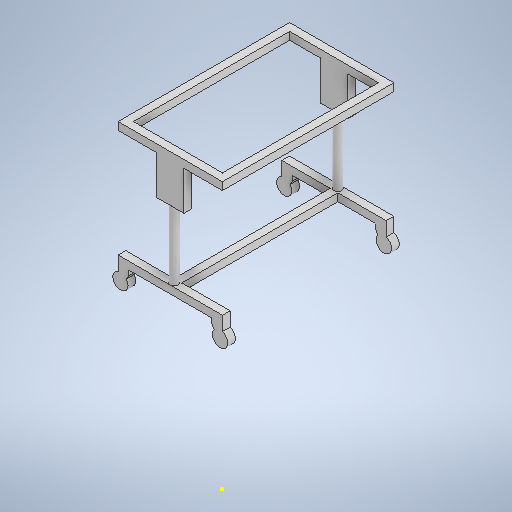
# Autodesk Inventor part: Human-Subject-Cart
Saved by Autodesk Inventor 2025.1 (Build 291241000, 241)
## iProperties
Created: 2025-01-22
Part Number: Human-Subject-Cart
Material: Generic
Document SubType Name: Modeling
Designer: jmarvel
Density: 1 g/cm^3
Appearance: Default
Author: jmarvel
Autodesk Inventor part; units mm, degrees
ref_plane "YZ Plane" through (0, 0, 0) normal (1, 0, 0) x (0, 1, 0)
ref_plane "XZ Plane" through (0, 0, 0) normal (0, 1, 0) x (-1, 0, 0)
ref_plane "XY Plane" through (0, 0, 0) normal (0, 0, 1) x (1, 0, 0)
sketch "Sketch1" plane through (0, 0, 0) normal (0, 1, 0) x (-1, 0, 0)
  line L0 (0, 0) -> (680, 0)
  line L1 (680, 0) -> (680, -1118)
  line L2 (680, -1118) -> (0, -1118)
  line L3 (0, -1118) -> (0, 0)
  dimension "d0" = 680
  dimension "d1" = 1118
  constraints: 8 end point, 2 parallel, 1 horizontal, 1 perpendicular
  measures "d0" distance of L1.end L2.end
  measures "d1" distance of L0.end L1.end
extrude "Extrusion1" add sketch "Sketch1" along normal blind 50
sketch "Sketch2" plane through (0, 50, 0) normal (0, 1, 0) x (1, 0, 0)
  line L0 (-50, 50) -> (-630, 50)
  line L1 (-630, 50) -> (-630, 1068)
  line L2 (-630, 1068) -> (-50, 1068)
  line L3 (-50, 1068) -> (-50, 50)
  point P0 (0, 0)
  dimension "d4" = 580
  dimension "d5" = 1018
  constraints: 8 end point, 2 parallel, 1 horizontal, 1 perpendicular
  measures "d4" distance of L1.end L2.end
  measures "d5" distance of L0.end L1.end
extrude "Extrusion2" cut sketch "Sketch2" against normal blind 50
sketch "Sketch3" plane through (0, 50, 0) normal (0, 1, 0) x (1, 0, 0)
  point P0 (0, 0)
sketch "Sketch4" plane through (0, 50, 0) normal (0, 1, 0) x (1, 0, 0)
  line L0 (-680, 0) -> (0, 0) projected
  line L1 (-251, 0) -> (-429, 0)
  line L2 (-429, 0) -> (-429, 50)
  line L3 (-429, 50) -> (-251, 50)
  line L4 (-251, 50) -> (-251, 0)
  dimension "d8" = 178
  dimension "d9" = 50
  constraints: 8 end point, 2 parallel, 1 horizontal, 1 perpendicular, 1 point on line
  measures "d8" distance of L2.end L3.end
  measures "d9" distance of L1.end L2.end
extrude "Extrusion3" add sketch "Sketch4" along normal blind 254
sketch "Sketch5" plane through (0, 50, 0) normal (0, 1, 0) x (1, 0, 0)
  line L0 (0, 1118) -> (-680, 1118) projected
  line L1 (-630, 1068) -> (-50, 1068) projected
  line L2 (-251, 1118) -> (-429, 1118)
  line L3 (-429, 1118) -> (-429, 1068)
  line L4 (-429, 1068) -> (-251, 1068)
  line L5 (-251, 1068) -> (-251, 1118)
  point P0 (0, 0)
  dimension "d12" = 178
  constraints: 8 end point, 2 parallel, 2 point on line, 1 horizontal, 1 perpendicular
  measures "d12" distance of L4.end L3.end
extrude "Extrusion4" add sketch "Sketch5" along normal blind 254
sketch "Sketch6" plane through (0, 304, 0) normal (0, 1, 0) x (1, 0, 0)
  circle A0 centre (-340, 25) radius 25
  point P0 (0, 0)
  dimension "d15" = 50
  constraints: 1 centre point
  measures "d15" diameter of A0
extrude "Extrusion5" add sketch "Sketch6" along normal blind 450
sketch "Sketch7" plane through (0, 304, 0) normal (0, 1, 0) x (1, 0, 0)
  circle A0 centre (-340, 1093) radius 25
  point P0 (0, 0)
  dimension "d18" = 50
  constraints: 1 centre point
  measures "d18" diameter of A0
extrude "Extrusion6" add sketch "Sketch7" along normal blind 450
sketch "Sketch8" plane through (-340, 754, -25) normal (0, 1, 0) x (1, 0, 0)
  line L0 (-340, -25) -> (340, -25) projected
  line L1 (25, -25) -> (-25, -25)
  line L2 (-25, -25) -> (-25, 1093)
  line L3 (-25, 1093) -> (25, 1093)
  line L4 (25, 1093) -> (25, -25)
  dimension "d21" = 50
  dimension "d22" = 1118
  constraints: 8 end point, 2 parallel, 1 horizontal, 1 perpendicular, 1 point on line
  measures "d21" distance of L2.end L3.end
  measures "d22" distance of L1.end L2.end
extrude "Extrusion7" add sketch "Sketch8" along normal blind 50
sketch "Sketch9" plane through (-315, 754, -25) normal (1, 0, 0) x (0, 0, -1)
  line L0 (0, 0) -> (-25, 0) projected
  line L1 (-25, 0) -> (25, 0)
  line L2 (25, 0) -> (25, 50)
  line L3 (25, 50) -> (-25, 50)
  line L4 (-25, 50) -> (-25, 0)
  point P0 (-25, -754)
  dimension "d25" = 50
  dimension "d26" = 50
  constraints: 8 end point, 2 parallel, 1 horizontal, 1 perpendicular
  measures "d25" distance of L3.end L2.end
  measures "d26" distance of L2.end L1.end
extrude "Extrusion8" add sketch "Sketch9" along normal blind 315
sketch "Sketch10" plane through (-315, 754, -1093) normal (1, 0, 0) x (0, 0, -1)
  line L0 (25, 0) -> (25, 50) projected
  line L1 (25, 0) -> (-25, 0)
  line L2 (-25, 0) -> (-25, 50)
  line L3 (-25, 50) -> (25, 50)
  line L4 (25, 50) -> (25, 0)
  point P0 (-1093, -754)
  dimension "d29" = 50
  dimension "d30" = 50
  constraints: 8 end point, 2 parallel, 1 horizontal, 1 perpendicular
  measures "d29" distance of L2.end L3.end
  measures "d30" distance of L1.end L2.end
extrude "Extrusion9" add sketch "Sketch10" along normal blind 315
sketch "Sketch11" plane through (-365, 754, -1093) normal (-1, 0, 0) x (0, 0, 1)
  line L0 (-25, 50) -> (1093, 50) projected
  line L1 (-25, 50) -> (25, 50)
  line L2 (25, 50) -> (25, 0)
  line L3 (25, 0) -> (-25, 0)
  line L4 (-25, 0) -> (-25, 50)
  point P0 (1093, -754)
  dimension "d33" = 50
  dimension "d34" = 50
  constraints: 8 end point, 2 parallel, 1 horizontal, 1 perpendicular
  measures "d33" distance of L2.end L3.end
  measures "d34" distance of L1.end L2.end
extrude "Extrusion10" add sketch "Sketch11" along normal blind 315
sketch "Sketch12" plane through (-365, 754, -25) normal (-1, 0, 0) x (0, 0, 1)
  line L0 (-1043, 50) -> (25, 50) projected
  line L1 (25, 50) -> (-25, 50)
  line L2 (-25, 50) -> (-25, 0)
  line L3 (-25, 0) -> (25, 0)
  line L4 (25, 0) -> (25, 50)
  point P0 (25, -754)
  dimension "d37" = 50
  dimension "d38" = 50
  constraints: 8 end point, 2 parallel, 1 horizontal, 1 perpendicular
  measures "d37" distance of L3.end L2.end
  measures "d38" distance of L2.end L1.end
extrude "Extrusion11" add sketch "Sketch12" along normal blind 315
sketch "Sketch13" plane through (0, 754, -1118) normal (0, 0, -1) x (-1, 0, 0)
  line L0 (680, 0) -> (680, 50) projected
  line L1 (680, 50) -> (610, 50)
  line L2 (610, 50) -> (610, 80.718)
  line L3 (650, 150) -> (680, 150)
  line L4 (680, 150) -> (680, 50)
  line L5 (0, 50) -> (70, 50)
  line L6 (70, 50) -> (70, 80.718)
  line L7 (30, 150) -> (0, 150)
  line L8 (0, 150) -> (0, 50)
  line L9 (650, 150) -> (610, 80.718)
  line L10 (650, 150) -> (680, 150) construction
  line L11 (30, 150) -> (70, 80.718)
  point P0 (0, -754)
  constraints: 22 end point, 4 parallel, 3 horizontal, 2 perpendicular, 1 point on line
extrude "Extrusion12" add sketch "Sketch13" against normal blind 1118
sketch "Sketch14" plane through (0, 754, -25) normal (1, 0, 0) x (0, 0, -1)
  line L0 (25, 50) -> (1043, 50) projected
  line L1 (1043, 50) -> (25, 50)
  line L2 (25, 50) -> (25, 150)
  line L3 (25, 150) -> (1043, 150)
  line L4 (1043, 150) -> (1043, 50)
  point P0 (-25, -754)
  constraints: 8 end point, 2 parallel, 1 horizontal, 1 perpendicular
extrude "Extrusion13" cut sketch "Sketch14" against normal blind 1118
sketch "Sketch15" plane through (-340, 754, 0) normal (0, 0, 1) x (1, 0, 0)
  circle A0 centre (325, 140) radius 50
  circle A1 centre (-325, 140) radius 50
  line L0 (340, 0) -> (340, 150) projected
  line L1 (340, 0) -> (340, 150) projected
  line L2 (0, 0) -> (-340, 0) projected
  line L3 (0, 0) -> (340, 0) projected
  line L4 (340, 0) -> (340, 150) projected
  line L5 (340, 150) -> (310, 150) projected
  line L6 (310, 150) -> (270, 80.718) projected
  line L7 (270, 80.718) -> (270, 50) projected
  line L8 (270, 50) -> (-270, 50) projected
  line L9 (-270, 50) -> (-270, 80.718) projected
  line L10 (-270, 80.718) -> (-310, 150) projected
  line L11 (-310, 150) -> (-340, 150) projected
  line L12 (-340, 0) -> (-340, 150) projected
  point P0 (340, -754)
  point P1 (340, 92.303)
  point P2 (286.0942, 108.594)
  constraints: 2 centre point
extrude "Extrusion14" add sketch "Sketch15" against normal blind 1118 contours A0 L0 L5 L6 | L12 L11 L10 A1 | A1 L10 L11 L12 picked at (325.7082, 163.3183)
move or copy body "Rotate1" bodies to move or copy 1 copy no rotation origin (0, 0, 0) rotation axis (1, 0, 0) rotation angle 180 translate (0, 1788, -1118)
sketch "Sketch16" plane through (0, 1034, 0) normal (1, 0, 0) x (0, 0, -1)
  line L0 (50, 0) -> (50, -92.303) projected
  line L1 (50, -72.2577) -> (1068, -72.2577)
  line L2 (1068, -72.2577) -> (1068, -234.0796)
  line L3 (1068, -234.0796) -> (50, -234.0796)
  line L4 (50, -234.0796) -> (50, -72.2577)
  point P0 (0, -1034)
  dimension "d58" = 1018
  constraints: 8 end point, 2 parallel, 1 horizontal, 1 perpendicular, 1 point on line
  measures "d58" distance of L2.end L3.end
extrude "Extrusion15" cut sketch "Sketch16" against normal blind 1118
sketch "Sketch17" plane through (-680, 1034, -1118) normal (-1, 0, 0) x (0, 0, 1)
  line L0 (1118, -80.718) -> (1068, -80.718) projected
  line L1 (1068, -80.718) -> (50, -80.718)
  line L2 (50, -80.718) -> (50, -329.635)
  line L3 (50, -329.635) -> (1068, -329.635)
  line L4 (1068, -329.635) -> (1068, -80.718)
  point P0 (1118, -1034)
  dimension "d61" = 1018
  constraints: 8 end point, 2 parallel, 1 horizontal, 1 perpendicular
  measures "d61" distance of L3.end L2.end
extrude "Extrusion16" cut sketch "Sketch17" against normal blind 1118
body "Solid1"
